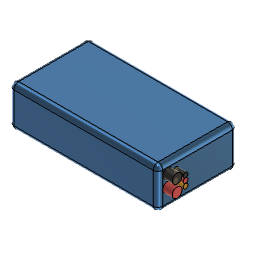
Battary 7.4 v (Autodesk Fusion 360 design; units mm, degrees)
Autodesk Fusion 360 part; units mm, degrees
sketch "Sketch1" plane through (0, 0, 0) normal (0, 0, 1) x (1, 0, 0)
  line L0 (-25, 0) -> (-25, 33)
  line L1 (-25, 33) -> (37, 33)
  line L2 (-25, 0) -> (37, 0)
  line L3 (37, 0) -> (37, 33)
  dimension "d1" = 33
  dimension "d2" = 62
  dimension "d3" = 62
  constraint vertical L0
  constraint perpendicular L0 L1
  constraint perpendicular L0 L2
  measures "d1" distance of L0.start L0.end
  measures "d2" distance of L0.end L1.end
  measures "d3" distance of L0.start L2.end
extrude "Extrude1" add sketch "Sketch1" along normal blind 17 makes body 1
fillet "Fillet1" radius 2 4 edges at (-25, 0, 8.5) (-25, 33, 8.5) (37, 0, 8.5) (37, 33, 8.5) on bodies 1
fillet "Fillet2" radius 2 16 edges at (-24.4142, 0.5858, 17) (6, 0, 17) (36.4142, 0.5858, 17) (37, 16.5, 17) (36.4142, 32.4142, 17) (6, 33, 17) (-24.4142, 32.4142, 17) (-25, 16.5, 17) (-24.4142, 32.4142, 0) (6, 33, 0) (36.4142, 32.4142, 0) (37, 16.5, 0) (36.4142, 0.5858, 0) (6, 0, 0) (-24.4142, 0.5858, 0) (-25, 16.5, 0) on bodies 1
sketch "Sketch2" plane through (37, 0, 0) normal (1, 0, 0) x (0, 1, 0)
  line L0 (2, 2) -> (31, 2)
  line L1 (31, 2) -> (31, 15)
  line L2 (31, 15) -> (2, 15)
  line L3 (2, 15) -> (2, 2)
  circle A0 centre (4, 13) radius 2
  circle A1 centre (4, 8) radius 2
  circle A2 centre (7.5, 12.5) radius 1
  circle A3 centre (7.5, 10.5) radius 1
  circle A4 centre (7.5, 8.5) radius 1
  constraint tangent L3 A0
  constraint tangent L3 A1
extrude "Extrude2" add sketch "Sketch2" along normal blind 4 separate body contours A1 | A0 | A2 | A4 | A3 makes body 2 at (39.6667, 5.9901, 13.1991) makes body 3 at (39.6667, 5.9901, 8.1991) makes body 4 at (39.6667, 7.4502, 9.5012)
